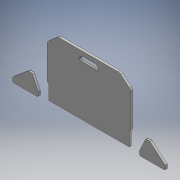
# Autodesk Inventor part: stand
Saved by Autodesk Inventor 2016 (Build 200138000, 138)
## iProperties
Created: 2016-10-17
Part Number: stand
Material: Generic
Document SubType Name: Modeling
Designer: rawrdong
Density: 1 g/cm^3
Appearance: Default
Author: rawrdong
Autodesk Inventor part; units mm, degrees
ref_plane "YZ Plane" through (0, 0, 0) normal (1, 0, 0) x (0, 1, 0)
ref_plane "XZ Plane" through (0, 0, 0) normal (0, 1, 0) x (-1, 0, 0)
ref_plane "XY Plane" through (0, 0, 0) normal (0, 0, 1) x (1, 0, 0)
sketch "Sketch1" plane through (0, 0, 0) normal (0, 1, 0) x (-1, 0, 0)
  line L0 (0, 508) -> (260.2597, 508)
  line L1 (260.2597, 508) -> (355.6, 428)
  line L2 (355.6, 428) -> (355.6, 130)
  line L3 (343.1, 0) -> (0, 0)
  line L4 (-60, 448) -> (60, 448) construction
  line L5 (0, 468) -> (60, 468)
  line L6 (80, 428) -> (0, 428)
  line L7 (0, 0) -> (0, 428)
  line L8 (0, 468) -> (0, 508)
  line L9 (343.1, 0) -> (343.1, 123.65)
  line L10 (343.1, 130) -> (355.6, 130)
  arc A0 (343.1, 130) -> (343.1, 123.65) centre (343.1, 126.825) ccw
  line L11 (60, 468) -> (80, 451.218)
  line L12 (80, 451.218) -> (80, 428)
  point P0 (0, 448)
  dimension "d0" = 40
  dimension "d1" = 40
  dimension "d2" = 140
  dimension "d4" = 120
  dimension "d5" = 508
  dimension "d8" = 12.5
  dimension "d9" = 355.6
  dimension "d23" = 130
  dimension "d25" = 6.35
  dimension "d28" = 20
  constraints: 28 end point, 6 perpendicular, 4 parallel, 4 vertical, 2 point on circle, 2 vertical alignment, 1 centre point, 1 collinear, 1 horizontal alignment, 1 midpoint, 1 point on line, 1 tangent
  measures "d0" distance between parallel lines of L6 L5
  measures "d1" distance between parallel lines of L0 L5
  measures "d2" angle of L0 L1
  measures "d4" distance of L4.start L4.end
  measures "d5" distance between parallel lines of L3 L0
  measures "d8" distance between parallel lines of L2 L9
  measures "d9" distance between parallel lines of L7 L2
  measures "d23" distance of L3.start L10.start
  measures "d25" diameter of A0
  measures "d28" distance from line of L5.end L12
extrude "Extrusion1" add sketch "Sketch1" along normal blind 17.5
mirror "Mirror1" about plane through (0, 0, 428) normal (1, 0, 0) of "Extrusion1"
sketch "Sketch2" plane through (0, 0, 0) normal (0, 1, 0) x (-1, 0, 0)
  line L0 (430.6, -20) -> (650.6, -20)
  line L1 (516.85, 130) -> (484.35, 130)
  line L2 (500.6, 130) -> (500.6, -20) construction
  line L3 (516.85, 130) -> (650.6, 17.7704)
  line L4 (650.6, 17.7704) -> (650.6, -20)
  line L5 (430.6, -20) -> (430.6, 17.7704)
  line L6 (430.6, 17.7704) -> (484.35, 130)
  point P0 (0, 0)
  point P1 (355.6, 130)
  point P2 (343.1, 0)
  dimension "d10" = 32.5
  dimension "d11" = 70
  dimension "d12" = 150
  dimension "d13" = 75
  dimension "d14" = 20
  dimension "d29" = 140
  constraints: 14 end point, 3 vertical, 2 horizontal alignment, 1 horizontal, 1 midpoint, 1 parallel, 1 point on line
  measures "d10" distance of L1.start L1.end
  measures "d11" distance from line of L0.start L2
  measures "d12" distance from line of L0.end L2
  measures "d13" horizontal distance of point (355.6, 130) L0.start
  measures "d14" distance from line of point (343.1, 0) L0
  measures "d29" angle of L1 L3
extrude "Extrusion2" add sketch "Sketch2" along normal blind 17.5 separate body
sketch "Sketch3" plane through (0, 17.5, 0) normal (0, 1, 0) x (1, 0, 0)
  line L0 (-430.6, 20) -> (-650.6, 20) projected
  line L1 (-516.85, -130) -> (-484.35, -130) construction
  line L2 (-484.35, -130) -> (-516.85, -130)
  line L3 (-500.6, -130) -> (-500.6, -37.4483) construction
  line L4 (-491.5325, -130) -> (-509.6675, -130)
  line L5 (-509.6675, -130) -> (-509.6675, 0)
  line L6 (-509.6675, 0) -> (-491.5325, 0)
  line L7 (-491.5325, 0) -> (-491.5325, -130)
  circle A0 centre (-494.7075, 0) radius 3.175
  circle A1 centre (-506.4925, 0) radius 3.175
  point P0 (0, 0)
  point P1 (-343.1, 0)
  dimension "d24" = 6.35
  dimension "d19" = 18.135
  constraints: 12 end point, 3 equal length, 3 horizontal alignment, 3 point on line, 1 horizontal, 1 midpoint, 1 perpendicular, 1 vertical, 5 other
  measures "d19" distance between parallel lines of L5 L7
extrude "Extrusion3" cut sketch "Sketch3" against normal blind 5 bodies 2
fillet "Fillet1" radius 30 4 edges at (355.6, 8.75, 428) (260.2597, 8.75, 508) (-260.2597, 8.75, 508) (-355.6, 8.75, 428)
fillet "Fillet1" radius 10 9 edges at (-80, 8.75, 451.218) (-80, 8.75, 428) (80, 8.75, 428) (80, 8.75, 451.218) (-650.6, 8.75, 17.7704) (-430.6, 8.75, -20) (-650.6, 8.75, -20) (-516.85, 8.75, 130) (-484.35, 8.75, 130)
fillet "Fillet1" radius 20 3 edges at (60, 8.75, 468) (-60, 8.75, 468) (-430.6, 8.75, 17.7704)
mirror "Mirror2" about plane through (0, 0, 0) normal (1, 0, 0) bodies 2
equation "\"d8\" = mt - inset"
equation "\"d6\" = mt"
equation "\"d15\" = mt"
equation "\"d17\" = inset"
equation "\"mt\" = 17.5"
equation "\"inset\" = 5"
